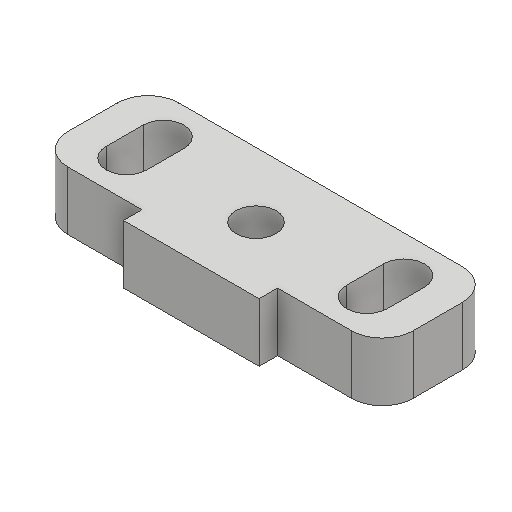
# Autodesk Inventor part: 3DP_ABS_Extruder_Tensioning_Arm_Screw_Mount
Saved by Autodesk Inventor 2026.1 (Build 301233000, 233)
## iProperties
Created: 2016-01-23
Part Number: 3DP_ABS_Extruder_Tensioning_Arm_Screw_Mount
Material: Ogólny
Document SubType Name: Modeling
Designer: Andrzej
Density: 1 g/cm^3
Appearance: Default
Mass: 1.03518 g
Surface Area: 9.85217 cm^2
Volume: 1.03518 cm^3
Author: Andrzej
Autodesk Inventor part; units mm, degrees
ref_plane "YZ Plane" through (0, 0, 0) normal (1, 0, 0) x (0, 1, 0)
ref_plane "XZ Plane" through (0, 0, 0) normal (0, 1, 0) x (-1, 0, 0)
ref_plane "XY Plane" through (0, 0, 0) normal (0, 0, 1) x (1, 0, 0)
sketch "Szkic1" plane through (0, 0, 0) normal (0, 0, 1) x (1, 0, 0)
  line L0 (-9.6574, 2.8417) -> (18.3426, 2.8417)
  line L1 (18.3426, 2.8417) -> (18.3426, -6.1583)
  line L2 (18.3426, -6.1583) -> (-9.6574, -6.1583)
  line L3 (-9.6574, -6.1583) -> (-9.6574, 2.8417)
  line L4 (-1.1574, -6.1583) -> (-1.1574, -7.6583)
  line L5 (-1.1574, -7.6583) -> (9.8426, -7.6583)
  line L6 (9.8426, -7.6583) -> (9.8426, -6.1583)
  point P0 (0, 0)
  point P1 (4.3426, -2.4083)
  dimension "d0" = 28
  dimension "d1" = 9
  dimension "d2" = 1.5
  dimension "d3" = 11
  dimension "d4" = 8.5
  dimension "d20" = 14
  dimension "d21" = 10.5
  dimension "d22" = 5.25
  constraints: 14 end point, 5 perpendicular, 2 point on line, 1 horizontal, 1 parallel
  measures "d0" distance of L0.start L0.end
  measures "d1" distance of L0.end L1.end
  measures "d2" distance of L4.start L4.end
  measures "d3" distance between parallel lines of L6 L4
  measures "d4" distance between parallel lines of L3 L4
  measures "d20" distance from line of L3 point (4.343, -2.408)
  measures "d21" distance between parallel lines of L0 L5
  measures "d22" distance from line of L5 point (4.343, -2.408)
extrude "Wyciągnięcie proste1" add sketch "Szkic1" along normal blind 4.75
sketch "Szkic2" plane through (0, 0, 4.75) normal (0, 0, 1) x (1, 0, 0)
  line L0 (-9.6574, -6.1583) -> (-1.1574, -6.1583) projected
  line L1 (9.8426, -6.1583) -> (18.3426, -6.1583) projected
  line L2 (18.3426, 2.8417) -> (-9.6574, 2.8417) projected
  line L3 (-9.6574, 2.8417) -> (-9.6574, -6.1583) projected
  line L4 (18.3426, -6.1583) -> (18.3426, 2.8417) projected
  line L5 (14.0926, -3.1583) -> (14.0926, -0.1583) construction
  line L6 (15.7426, -3.1583) -> (15.7426, -0.1583)
  line L7 (12.4426, -0.1583) -> (12.4426, -3.1583)
  arc A0 (12.4426, -3.1583) -> (15.7426, -3.1583) centre (14.0926, -3.1583) ccw
  arc A1 (15.7426, -0.1583) -> (12.4426, -0.1583) centre (14.0926, -0.1583) ccw
  line L8 (-5.4074, -3.1583) -> (-5.4074, -0.1583) construction
  line L9 (-3.7574, -3.1583) -> (-3.7574, -0.1583)
  line L10 (-7.0574, -0.1583) -> (-7.0574, -3.1583)
  arc A2 (-7.0574, -3.1583) -> (-3.7574, -3.1583) centre (-5.4074, -3.1583) ccw
  arc A3 (-3.7574, -0.1583) -> (-7.0574, -0.1583) centre (-5.4074, -0.1583) ccw
  point P0 (0, 0)
  point P1 (-5.4074, -1.6583)
  point P2 (14.0926, -1.6583)
  dimension "d7" = 4.5
  dimension "d8" = 4.5
  dimension "d9" = 9
  dimension "d10" = 8.5
  dimension "d11" = 4.25
  dimension "d12" = 4.25
  dimension "d13" = 1.5
  dimension "d14" = 3.3
  dimension "d15" = 1.5
  dimension "d16" = 3.3
  constraints: 16 end point, 8 point on circle, 8 tangent, 4 centre point, 3 parallel, 2 midpoint, 1 vertical
  measures "d7" distance from line of L0 point (-5.407, -1.658)
  measures "d8" distance from line of L1 point (14.093, -1.658)
  measures "d9" distance between parallel lines of L0 L2
  measures "d10" distance of L0.start L0.end
  measures "d11" distance from line of L3 point (-5.407, -1.658)
  measures "d12" distance from line of L4 point (14.093, -1.658)
  measures "d13" distance of point (14.093, -1.658) L5.end
  measures "d14" diameter of A1
  measures "d15" distance of point (-5.407, -1.658) L8.end
  measures "d16" diameter of A3
extrude "Wyciągnięcie proste2" cut sketch "Szkic2" against normal blind 10
fillet "Zaokrąglenie1" radius 2.5 4 edges at (-9.6574, 2.8417, 2.375) (-9.6574, -6.1583, 2.375) (18.3426, -6.1583, 2.375) (18.3426, 2.8417, 2.375)
hole "Otwór1" at (4.3426, -2.4083, 0) direction (0, 0, 1) diameter 3.25 end through all
equation "\"d4\" = -0.5 * d3 + 0.5 * d0"
equation "\"d20\" = 0.5 * d0"
equation "\"d22\" = 0.5 * d21"
equation "\"d7\" = 0.5 * d9"
equation "\"d8\" = d7"
equation "\"d11\" = 0.5 * d10"
equation "\"d12\" = d11"
